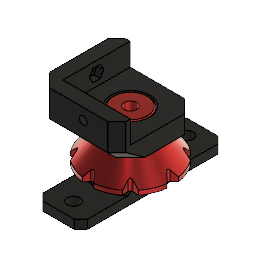
Build Plate Support Assy (Autodesk Fusion 360 design; units mm, degrees)
description: Build Plate Support Assy
part number: VK-A-BPS
Autodesk Fusion 360 part; units mm, degrees
sketch "Sketch4" plane through (0, 0, 0) normal (0, 0, 1) x (1, 0, 0)
  line L0 (0, 0) -> (20, 0)
  line L1 (20, 0) -> (20, 64)
  line L2 (20, 64) -> (0, 64)
  line L3 (0, 64) -> (0, 0)
  dimension "d47" = 20
  dimension "d48" = 64
  constraint horizontal L0
  constraint vertical L1
  constraint horizontal L2
  constraint vertical L3
  constraint coincident L0.start L3.end
  measures "d47" distance of L0.start L0.end
  measures "d48" distance of L0.start L2.end
extrude "Extrude11" add sketch "Sketch4" along normal blind 4 makes body 1
sketch "Sketch5" plane through (0, 0, 4) normal (0, 0, 1) x (-1, 0, 0)
  line L0 (-20, -64) -> (0, -64)
  line L1 (-20, 0) -> (-20, -64)
  line L2 (0, 0) -> (-20, 0)
  line L3 (0, -64) -> (0, 0)
  line L4 (-10, -64) -> (-10, 0) construction
  circle A0 centre (-10, -32) radius 2.75
  line L5 (-14, -29.6906) -> (-14, -34.3094)
  line L6 (-14, -34.3094) -> (-10, -36.6188)
  line L7 (-10, -36.6188) -> (-6, -34.3094)
  line L8 (-6, -34.3094) -> (-6, -29.6906)
  line L9 (-6, -29.6906) -> (-10, -27.3812)
  line L10 (-10, -27.3812) -> (-14, -29.6906)
  circle A1 centre (-10, -32) radius 7 construction
  circle A2 centre (-10, -32) radius 10
  point P0 (-10, -32)
  dimension "d51" = 5.5
  dimension "d52" = 8
  dimension "d55" = 2.5
  dimension "d718" = 20
  dimension "d719" = 3
  constraint midpoint L0 L4.start
  constraint midpoint L2 L4.end
  constraint midpoint L4 P0
  constraint coincident P0 A0.centre
  constraint vertical L5
  constraint concentric A1 A2
  measures "d51" diameter of A0
  measures "d52" distance of L6 L9
  measures "d718" diameter of A2
  measures "d719" distance of A1 A2
extrude "Extrude12" add sketch "Sketch5" along normal blind 3 contours A2 | L5 L6 L7 L8 L9 L10 bodies 1
extrude "Extrude17" cut sketch "Sketch5" against normal blind 7 contours A0 | L5 L6 L7 L8 L9 L10 bodies 1
sketch "Sketch17" plane through (0, 0, 7) normal (0, 0, 1) x (-1, 0, 0)
  circle A0 centre (-10, -32) radius 2.75
  circle A1 centre (-10, -32) radius 10
  circle A2 centre (-10, -32) radius 7
  dimension "d720" = 3
  constraint concentric A0 A2
  measures "d720" distance of A1 A2
extrude "Extrude31" add sketch "Sketch17" along normal blind 7 contours A1 bodies 1
chamfer "Chamfer7" distance 3 distance2 3 4 edges at (20, 64, 2) (20, 0, 2) (0, 0, 2) (0, 64, 2) measured on face at (20, 32, 1.3333) measured on face at (6.6667, 0, 2.6667) measured on face at (0, 32, 1.3333) measured on face at (13.3333, 64, 2.6667) on bodies 1
sketch "Sketch18" plane through (0, 0, 4) normal (0, 0, 1) x (-1, 0, 0)
  line L0 (-3, -64) -> (0, -61)
  line L1 (0, -61) -> (0, -3)
  line L2 (0, -3) -> (-3, 0)
  line L3 (-17, 0) -> (-20, -3)
  line L4 (-20, -3) -> (-20, -61)
  line L5 (-20, -61) -> (-17, -64)
  circle A0 centre (-10, -32) radius 2.75
  line L6 (-17, -64) -> (-3, -64)
  line L7 (-3, 0) -> (-17, 0)
  line L8 (-10, -57.25) -> (-10, -6.75) construction
  circle A1 centre (-10, -6.75) radius 2.75 construction
  dimension "d726" = 6.75
  dimension "d1087" = 5.5
  dimension "d1088" = 4.25
  constraint parallel L4 L8
  constraint midpoint A0.centre L8
  constraint coincident L8.end A1.centre
  measures "d726" distance of L7 L8.end
  measures "d1087" diameter of A1
hole "Hole1" at (10, 57.25, 4) at (10, 6.75, 4) direction (0, 0, -1) diameter 5.5 depth 17 tip angle 118 bodies 1
chamfer "Chamfer20" distance 5 angle 45 2 edges at (10, 22, 4) (10, 42, 4) on bodies 1
copy_body "Body->Comp2" bodies 1 removing the originals makes body 2 in component "Bed Support Bracket"
sketch "Sketch1" plane through (0, 0, 14) normal (0, 0, 1) x (-1, 0, 0) in component "Bed Thumb Screw"
  circle A0 centre (-10, -32) radius 2.75
  circle A1 centre (-10, -32) radius 19
  circle A2 centre (-10, -32) radius 6.5
  circle A3 centre (-10, -32) radius 7 construction
  circle A4 centre (-10, -32) radius 13 construction
  point P0 (-10, -32)
  dimension "d741" = 38
  dimension "d747" = 0.5
  dimension "d793" = 0
  dimension "d794" = 0
  dimension "d795" = 0
  dimension "d796" = 0
  dimension "d809" = 0
  dimension "d810" = 0
  dimension "d811" = 0
  dimension "d812" = 0
  dimension "d893" = 0
  dimension "d894" = 0
  dimension "d895" = 0
  dimension "d896" = 0
  dimension "d978" = 13.5
  dimension "d980" = 14
  dimension "d992" = 0
  dimension "d993" = 0
  dimension "d994" = 0
  dimension "d995" = 0
  dimension "d1016" = 26
  dimension "d1053" = 0
  dimension "d1054" = 0
  dimension "d1055" = 0
  dimension "d1056" = 0
  dimension "d1065" = 0
  dimension "d1066" = 0
  dimension "d1067" = 0
  dimension "d1068" = 0
  constraint coincident P0 A0.centre
  constraint concentric A0 A4
  constraint concentric A1 A4
  measures "d741" diameter of A1
  measures "d747" distance of A2 A3
  measures "d980" diameter of A3
  measures "d1016" diameter of A4
extrude "Extrude1" add sketch "Sketch1" against normal blind 7 separate body contours A2 makes body 3 in component "Bed Thumb Screw"
sketch "Sketch2" plane through (0, 0, 7) normal (0, 0, -1) x (1, 0, 0) in component "Bed Thumb Screw"
  circle A0 centre (10, -32) radius 2.75 construction
  circle A1 centre (10, -32) radius 6.5
  line L0 (14, -34.3094) -> (14, -29.6906)
  line L1 (14, -29.6906) -> (10, -27.3812)
  line L2 (10, -27.3812) -> (6, -29.6906)
  line L3 (6, -29.6906) -> (6, -34.3094)
  line L4 (6, -34.3094) -> (10, -36.6188)
  line L5 (10, -36.6188) -> (14, -34.3094)
  point P0 (10, -32)
  dimension "d781" = 8
  constraint coincident P0 A0.centre
  constraint vertical L0
  measures "d781" distance of L1 L4
extrude "Extrude9" cut sketch "Sketch2" against normal blind 4 contours L0 L1 L2 L3 L4 L5 bodies 3 in component "Bed Thumb Screw"
extrude "Extrude2" add sketch "Sketch1" along normal blind 8 contours A1 | A2 bodies 3 in component "Bed Thumb Screw"
sketch "Sketch7" plane through (0, 0, 14) normal (0, 0, -1) x (1, 0, 0) in component "Bed Thumb Screw"
  circle A0 centre (10, -32) radius 19
  circle A1 centre (10, -32) radius 12
  dimension "d1360" = 24
  constraint concentric A0 A1
  measures "d1360" diameter of A1
extrude "Extrude12'" add sketch "Sketch7" along normal blind 7 bodies 3 in component "Bed Thumb Screw"
chamfer "Chamfer1" distance 11 angle 50 1 edges at (27.7142, 38.8707, 22) measured on face at (-3.5024, 33.0806, 22) on bodies 3 in component "Bed Thumb Screw"
sketch "Sketch8" plane through (0, 0, 7) normal (0, 0, -1) x (1, 0, 0) in component "Bed Thumb Screw"
  circle A0 centre (10, -32) radius 19
  circle A1 centre (10, -32) radius 12
  circle A2 centre (10, -32) radius 19
  line L0 (10, -32) -> (10, -13) construction
  line L1 (7.5, -13.1652) -> (10, -16)
  line L2 (12.5, -13.1652) -> (10, -16)
  point P0 (10, -32)
  dimension "d1348" = 38
  dimension "d1352" = 3
  dimension "d1353" = 5
  constraint coincident P0 A0.centre
  constraint coincident A0 L0.end
  constraint vertical L0
  constraint coincident A2 L1.start
  constraint coincident L0 L1.end
  constraint coincident A0 L2.start
  constraint symmetric L0 L1.start L2.start
  measures "d1348" diameter of A0
  measures "d1352" distance of L0.end L1.end
  measures "d1353" distance of L1.start L2.start
extrude "Extrude13" cut sketch "Sketch8" against normal blind 9 contours A0 A2 L1 L2 picked at (10, -14.0123) bodies 3 in component "Bed Thumb Screw"
fillet "Fillet2" radius 1 1 edges at (10, 16, 9.733) on bodies 3 in component "Bed Thumb Screw"
pattern_circular "C-Pattern2" count 8 over 360 about axis through (10, 32, 7) along (0, 0, -1) of "Extrude13", "Fillet2" in component "Bed Thumb Screw"
extrude "Extrude10" add 1 faces at (14.8301, 28.0605, 22) along direction (0, 0, 1) blind 6 on bodies 3 bodies 3 in component "Bed Thumb Screw"
chamfer "Chamfer4" distance 0.5 angle 45 1 edges at (17.4586, 34.8929, 28) on bodies 3 in component "Bed Thumb Screw"
chamfer "Chamfer5" distance 2 angle 45 1 edges at (-1.1879, 27.6606, 7) on bodies 3 in component "Bed Thumb Screw"
sketch "Sketch1 (2)" plane through (0, 0, 28) normal (0, 0, 1) x (-1, 0, 0) in component "Bed Corner Support"
  line L0 (5, -47) -> (-25, -47)
  line L1 (-25, -47) -> (-25, -17)
  line L2 (-25, -17) -> (5, -17)
  line L3 (5, -17) -> (5, -47)
  line L4 (-25, -17) -> (5, -47) construction
  line L5 (5, -47) -> (11, -47)
  line L6 (11, -47) -> (11, -11)
  line L7 (11, -11) -> (-25, -11)
  line L8 (-25, -11) -> (-25, -17)
  circle A0 centre (-10, -32) radius 2.75
  circle A1 centre (-10, -32) radius 7.5 construction
  circle A2 centre (-10, -32) radius 8
  dimension "d750" = 30
  dimension "d751" = 30
  dimension "d758" = 6
  dimension "d759" = 6
  dimension "d805" = 0
  dimension "d806" = 0
  dimension "d807" = 0
  dimension "d808" = 0
  dimension "d905" = 0
  dimension "d906" = 0
  dimension "d907" = 0
  dimension "d908" = 0
  dimension "d917" = 0
  dimension "d918" = 0
  dimension "d919" = 0
  dimension "d920" = 0
  dimension "d988" = 0
  dimension "d989" = 0
  dimension "d990" = 0
  dimension "d991" = 0
  dimension "d1049" = 0
  dimension "d1050" = 0
  dimension "d1051" = 0
  dimension "d1052" = 0
  dimension "d1061" = 0
  dimension "d1062" = 0
  dimension "d1063" = 0
  dimension "d1064" = 0
  dimension "d1243" = 0
  dimension "d1244" = 0
  dimension "d1245" = 0
  dimension "d1246" = 0
  dimension "d1299" = 0
  dimension "d1300" = 0
  dimension "d1301" = 0
  dimension "d1302" = 0
  dimension "d1319" = 0
  dimension "d1320" = 0
  dimension "d1321" = 0
  dimension "d1322" = 0
  constraint horizontal L0
  constraint vertical L1
  constraint horizontal L2
  constraint vertical L3
  constraint perpendicular L3 L5
  constraint perpendicular L5 L6
  constraint perpendicular L1 L7
  constraint perpendicular L2 L8
  constraint midpoint L4 A0.centre
  measures "d750" distance of L0.start L0.end
  measures "d751" distance of L0.start L2.end
  measures "d758" distance of L1.end L7.end
  measures "d759" distance of L0.start L5.end
extrude "Extrude1'" add sketch "Sketch1 (2)" along normal blind 8 separate body contours L0 L1 L2 L3 | L2 L3 L5 L6 L7 L8 makes body 4 in component "Bed Corner Support"
chamfer "Chamfer3" distance 2 angle 40 1 edges at (17.4586, 29.1071, 28) measured on face at (2.0398, 32.7965, 30.6667) on bodies 4 in component "Bed Corner Support"
move_face "OffsetFaces1" offset -0.5 1 faces at (2.0398, 32.7965, 32) on bodies 4 in component "Bed Corner Support"
extrude "Extrude2'" add sketch "Sketch1 (2)" along normal blind 18 contours L2 L3 L5 L6 L7 L8 bodies 4 in component "Bed Corner Support"
sketch "Sketch19" plane through (0, 17, 0) normal (0, 1, 0) x (-1, 0, 0)
  line L0 (-25, 36) -> (5, 36)
  line L1 (5, 36) -> (5, 46)
  line L2 (5, 46) -> (-25, 46)
  line L3 (-25, 46) -> (-25, 36)
  line L4 (5, 46) -> (-25, 36) construction
  line L5 (-6.8246, 41) -> (-8.4123, 43.75)
  line L6 (-8.4123, 43.75) -> (-11.5877, 43.75)
  line L7 (-11.5877, 43.75) -> (-13.1754, 41)
  line L8 (-13.1754, 41) -> (-11.5877, 38.25)
  line L9 (-11.5877, 38.25) -> (-8.4123, 38.25)
  line L10 (-8.4123, 38.25) -> (-6.8246, 41)
  point P0 (-10, 41)
  dimension "d1092" = 5.5
  constraint coincident L1.end L2.start
  constraint coincident L0.start L3.end
  constraint midpoint L4 P0
  constraint horizontal L9
  measures "d1092" distance of L6 L9
extrude "Extrude4" cut sketch "Sketch19" against normal blind 3 contours L5 L6 L7 L8 L9 L10 bodies 4 in component "Bed Corner Support"
sketch "Sketch20" plane through (-5, 0, 0) normal (1, 0, 0) x (0, 1, 0)
  line L0 (17, 36) -> (47, 36)
  line L1 (47, 36) -> (47, 46)
  line L2 (47, 46) -> (17, 46)
  line L3 (17, 46) -> (17, 36)
  line L4 (17, 46) -> (47, 36) construction
  line L5 (33.5877, 38.25) -> (35.1754, 41)
  line L6 (35.1754, 41) -> (33.5877, 43.75)
  line L7 (33.5877, 43.75) -> (30.4123, 43.75)
  line L8 (30.4123, 43.75) -> (28.8246, 41)
  line L9 (28.8246, 41) -> (30.4123, 38.25)
  line L10 (30.4123, 38.25) -> (33.5877, 38.25)
  point P0 (32, 41)
  dimension "d1095" = 5.5
  constraint coincident L2.end L3.start
  constraint coincident L0.end L1.start
  constraint midpoint L4 P0
  constraint horizontal L10
  measures "d1095" distance of L7 L10
extrude "Extrude5" cut sketch "Sketch20" against normal blind 3 contours L5 L6 L7 L8 L9 L10 bodies 4 in component "Bed Corner Support"
hole "Hole5" at (10, 17, 41) direction (0, -1, 0) diameter 3.5 depth 10 tip angle 118 bodies 4 in component "Bed Corner Support"
hole "Hole6" at (-5, 32, 41) direction (-1, 0, 0) diameter 3.5 depth 10 tip angle 118 bodies 4 in component "Bed Corner Support"
chamfer "Chamfer2" distance 4 angle 45 2 edges at (25, 11, 37) (-11, 47, 37) on bodies 4 in component "Bed Corner Support"
chamfer "Chamfer4'" distance 6 angle 45 2 edges at (-11, 11, 37) (25, 47, 32) on bodies 4 in component "Bed Corner Support"
chamfer "Chamfer1'" distance 6 angle 45 5 edges at (8, 11, 28) (-11, 30, 28) (23, 13, 28) (-9, 45, 28) (-8, 14, 28) on bodies 4 in component "Bed Corner Support"
component "Bed Support Bracket" placed x (1, 0, 0) y (0, 1, 0) z (0, 0, 1) at (0, 0, 0)
component "Bed Thumb Screw" placed x (1, 0, 0) y (0, 1, 0) z (0, 0, 1) at (0, 0, 0)
component "Bed Corner Support" placed x (1, 0, 0) y (0, 1, 0) z (0, 0, 1) at (0, 0, -8)
equation "d751 = d750"
equation "d759 = d758"
named bodies: "Bottom Bed Support", "Bed Support Bracket", "Bed Thumb Screw", "Bed Corner Support"
